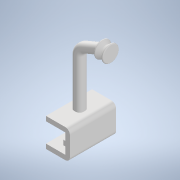
# Autodesk Inventor part: pully_holder
Saved by Autodesk Inventor 2021 (Build 250183000, 183)
## iProperties
Created: 2021-02-16
Part Number: pully_holder
Material: 일반
Document SubType Name: Modeling
Designer: jun85
Density: 1 g/cm^3
Appearance: 기본값
Author: jun85
Autodesk Inventor part; units mm, degrees
ref_plane "YZ Plane" through (0, 0, 0) normal (1, 0, 0) x (0, 1, 0)
ref_plane "XZ Plane" through (0, 0, 0) normal (0, 1, 0) x (-1, 0, 0)
ref_plane "XY Plane" through (0, 0, 0) normal (0, 0, 1) x (1, 0, 0)
sketch "스케치1" plane through (0, 0, 0) normal (0, 0, 1) x (1, 0, 0)
  line L0 (-10.5, -10.5) -> (10.5, -10.5)
  line L1 (10.5, -10.5) -> (10.5, 10.5)
  line L2 (10.5, 10.5) -> (-10.5, 10.5)
  line L3 (-10.5, 10.5) -> (-10.5, -10.5)
  line L4 (-10.5, -10.5) -> (10.5, 10.5) construction
  line L5 (10.5, -10.5) -> (-10.5, 10.5) construction
  line L6 (0, -37.38) -> (0, 115.78) projected
  line L7 (-15.5, 15.5) -> (15.5, 15.5)
  line L8 (15.5, 15.5) -> (15.5, -15.5)
  line L9 (15.5, -15.5) -> (-15.5, -15.5)
  line L10 (-15.5, -15.5) -> (-15.5, 15.5)
  line L11 (-4, 76.6432) -> (25, 88.9)
  line L12 (25, 88.9) -> (25, 78.9)
  line L13 (25, 78.9) -> (6, 70.8697)
  line L14 (-4, 15.5) -> (-4, 76.6432)
  line L15 (6, 15.5) -> (6, 70.8697)
  line L16 (-10.5, 10.5) -> (-10.5, 15.5)
  line L17 (-10.5, -10.5) -> (-10.5, -15.5)
  line L18 (10.5, 2.6) -> (8.5, 2.6)
  line L19 (8.5, 2.6) -> (8.5, -2.6)
  line L20 (8.5, -2.6) -> (10.5, -2.6)
  line L21 (10.5, -2.6) -> (10.5, 2.6)
  line L22 (-25.6, 0) -> (45.1, 0) projected
  line L23 (25, 83.9) -> (35, 83.9)
  line L24 (35, 83.9) -> (35, 93.9)
  line L25 (25, 93.9) -> (25, 83.9)
  line L26 (25, 93.9) -> (30, 89.9)
  line L27 (30, 89.9) -> (35, 93.9)
  line L28 (-4, 76.6432) -> (6, 70.8697) construction
  line L29 (25, 83.9) -> (25, 73.9)
  line L30 (25, 73.9) -> (30, 77.9)
  line L31 (30, 77.9) -> (35, 73.9)
  line L32 (35, 73.9) -> (35, 83.9)
  point P0 (0, 0)
  dimension "d2" = 21
  dimension "d3" = 5
  dimension "d9" = 10
  dimension "d10" = 10
  dimension "d11" = 4
  dimension "d12" = 5.2
  dimension "d13" = 2
  dimension "d15" = 10
  dimension "d16" = 6
  dimension "d17" = 10
  dimension "d27" = 30
  dimension "d28" = 60
  dimension "d29" = 6
  dimension "d30" = 77.9
  constraints: 62 end point, 9 parallel, 8 point on line, 6 equal length, 4 perpendicular, 4 vertical, 3 horizontal, 3 midpoint, 1 collinear, 4 other
  measures "d2" distance of L0.end L1.end
  measures "d3" distance between parallel lines of L2 L7
  measures "d9" distance of L11.end L12.end
  measures "d10" distance of L15.start L14.start
  measures "d11" distance from line of L6 L14.start
  measures "d12" distance of L18.end L19.end
  measures "d13" distance of L18.start L18.end
  measures "d15" distance of L23.end L24.end
  measures "d16" distance from line of L23 L26.end
  measures "d17" distance of L23.start L23.end
  measures "d27" distance from line of L6 L26.end
  measures "d28" angle of L14 L28
  measures "d29" distance from line of L30.end L23
  measures "d30" distance from line of L22 L30.end
extrude "돌출1" add sketch "스케치1" along normal mid plane 50 contours L0 L6 L9 L17 | L0 L1 L22 L8 L9 L6 | L16 L7 L6 L2 | L20 L19 L22 L1 | L6 L7 L8 L22 L1 L2 | L19 L18 L1 L22
extrude "돌출2" add sketch "스케치1" along normal mid plane 10 contours L7 L14 L11 L6 | L6 L11 L12 L13 L15 L7
revolve "회전1" add sketch "스케치1" angle 360 about axis through (25, 83.9, 0) along (1, 0, 0) contours L25 L26 L27 L24 L23 L12
fillet "모깎기1" radius 4 8 edges at (-4, 46.0716, 5) (10.5, 82.7716, 5) (15.5, 74.8848, 5) (6, 43.1848, 5) (15.5, 74.8848, -5) (6, 43.1848, -5) (10.5, 82.7716, -5) (-4, 46.0716, -5)
fillet "모깎기1" radius 1 2 edges at (25, 73.9, 0) (35, 73.9, 0)
fillet "모깎기1" radius 15 1 edges at (-4, 76.6432, 0)
fillet "모깎기1" radius 5 2 edges at (15.5, 15.5, 0) (15.5, -15.5, 0)
fillet "모깎기1" radius 5 1 edges at (6, 70.8697, 0)
fillet "모깎기1" radius 1 8 edges at (25, 88.9, 0) (25, 83.9, -5) (25, 78.9, 0) (25, 83.9, 5) (1, 15.5, -5) (-4, 15.5, 0) (1, 15.5, 5) (6, 15.5, 0)
sketch "스케치2" plane through (-10.5, -15.5, -25) normal (0, -1, 0) x (1, 0, 0)
  line L0 (0, 0) -> (0, 50) projected
  line L1 (21, 50) -> (0, 50) projected
  line L2 (21, 50) -> (21, 0) projected
  line L3 (0, 0) -> (21, 0) projected
  circle A0 centre (10.5, 39) radius 10.5 construction
  circle A1 centre (10.5, 39) radius 2.1
  circle A2 centre (10.5, 11) radius 2.1
  arc A3 (12.5, 19) -> (17.5, 24) centre (12.5, 24) ccw projected
  line L4 (17.5, 26) -> (17.5, 24) projected
  arc A4 (17.5, 26) -> (12.5, 31) centre (12.5, 26) ccw projected
  line L5 (10.5, 31) -> (12.5, 31) projected
  arc A5 (10.5, 31) -> (5.5, 26) centre (10.5, 26) ccw projected
  line L6 (5.5, 24) -> (5.5, 26) projected
  arc A6 (5.5, 24) -> (10.5, 19) centre (10.5, 24) ccw projected
  line L7 (12.5, 19) -> (10.5, 19) projected
  line L8 (21, 0) -> (21, 50) projected
  line L9 (0, 0) -> (21, 0) projected
  line L10 (0, 0) -> (0, 50) projected
  line L11 (21, 50) -> (0, 50) projected
  circle A7 centre (10.5, 39) radius 4
  circle A8 centre (10.5, 11) radius 4
  point P0 (10.5, 25)
  dimension "d33" = 4.2
  dimension "d34" = 11
  dimension "d35" = 11
  dimension "d36" = 8
  constraints: 5 centre point, 3 coincident, 2 equal radius, 2 tangent, 1 vertical alignment
  measures "d33" diameter of A1
  measures "d34" distance from line of A1.centre L1
  measures "d35" distance from line of L3 A2.centre
  measures "d36" diameter of A7
extrude "돌출3" cut sketch "스케치2" against normal blind 10 contours A1 | A2
extrude "돌출4" cut sketch "스케치2" against normal blind 2 contours A1 | A2 | A7 | A8
ref_plane "작업 평면1" through (-10.5, 0, -25) normal (0, -1, 0) x (1, 0, 0)
mirror "미러1" about plane through (-10.5, 0, -25) normal (0, -1, 0) of "돌출4", "돌출3"
